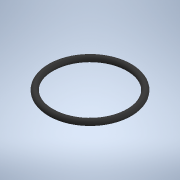
# Autodesk Inventor part: 16mm_o-ring
Saved by Autodesk Inventor 2020.2 (Build 242310000, 310)
## iProperties
Created: 2020-04-11
Part Number: 16mm_o-ring
Material: Rubber, Silicone
Document SubType Name: Modeling
Designer: agmlego
Mass: 0.0846675 g
Surface Area: 2.13335 cm^2
Volume: 0.067734 cm^3
Density: 1.25 g/cm^3
Appearance: Rubber - Black
Author: agmlego
Autodesk Inventor part; units mm, degrees
ref_plane "YZ Plane" through (0, 0, 0) normal (1, 0, 0) x (0, 1, 0)
ref_plane "XZ Plane" through (0, 0, 0) normal (0, 1, 0) x (-1, 0, 0)
ref_plane "XY Plane" through (0, 0, 0) normal (0, 0, 1) x (1, 0, 0)
sketch "Sketch1" plane through (0, 0, 0) normal (0, 0, 1) x (1, 0, 0)
  circle A0 centre (8.51, 0) radius 0.635
  line L0 (0, 6.8242) -> (0, -6.8242) construction
  line L1 (0, 0) -> (7.875, 0) construction
  dimension "d0" = 1.27
  dimension "d1" = 7.875
  constraints: 4 end point, 1 coincident, 1 horizontal alignment, 1 midpoint, 1 perpendicular, 1 point on line, 1 vertical, 2 other
  measures "d1" distance of L1.start L1.end
revolve "Revolution1" add sketch "Sketch1" angle 360 about axis through (0, 6.8242, 0) along (0, -1, 0)
body "Solid1"
